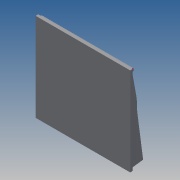
# Autodesk Inventor part: Bottom
Saved by Autodesk Inventor 2019 (Build 230136000, 136)
## iProperties
Created: 2022-10-28
Part Number: Bottom
Material: Generisch
Document SubType Name: Modeling
Designer: Dominik Schmidt
Density: 1 g/cm^3
Appearance: Vorgabe
Author: Dominik Schmidt
Autodesk Inventor part; units mm, degrees
ref_plane "YZ Plane" through (0, 0, 0) normal (1, 0, 0) x (0, 1, 0)
ref_plane "XZ Plane" through (0, 0, 0) normal (0, 1, 0) x (-1, 0, 0)
ref_plane "XY Plane" through (0, 0, 0) normal (0, 0, 1) x (1, 0, 0)
sketch "Skizze1" plane through (0, 0, 0) normal (0, 0, 1) x (1, 0, 0)
  line L0 (0, 0) -> (0, -76.060239)
  line L1 (0, -76.060239) -> (-35.95, -76.060239)
  line L2 (-45.45, -76.060239) -> (-81.4, -76.060239)
  line L3 (-81.4, -76.060239) -> (-81.4, 0)
  line L4 (-81.4, 0) -> (0, 0)
  line L5 (0, -76.060239) -> (-81.4, -76.060239)
  line L6 (-81.4, -76.060239) -> (-81.4, 0)
  line L7 (-81.4, 0) -> (0, 0)
  line L8 (0, 0) -> (0, -76.060239)
  constraints: 8 end point, 2 parallel, 1 horizontal, 1 perpendicular
extrude "Extrusion1" add sketch "Skizze1" along normal blind 2
sketch "Skizze2" plane through (0, 0, 0) normal (0, 0, -1) x (-1, 0, 0)
  point P0 (0, 0)
sketch "Skizze3" plane through (0, 0, 0) normal (0, 0, -1) x (-1, 0, 0)
  line L0 (35.95, -74.849731) -> (1.2, -74.849731)
  line L1 (80.2, -74.849731) -> (45.45, -74.849731)
  line L2 (49.95, -74.849731) -> (31.45, -74.849731)
  line L3 (31.45, -74.849731) -> (31.45, -50.349731)
  line L4 (31.45, -50.349731) -> (49.95, -50.349731)
  line L5 (49.95, -50.349731) -> (49.95, -74.849731)
  line L6 (81.4, 0) -> (81.4, -76.060239)
  line L7 (31.45, -50.349731) -> (29.45, -50.349731)
  line L8 (29.45, -50.349731) -> (29.45, -53.349731)
  line L9 (29.45, -53.349731) -> (31.45, -53.349731)
  line L10 (31.45, -53.349731) -> (31.45, -50.349731)
  line L11 (49.95, -50.349731) -> (51.95, -50.349731)
  line L12 (51.95, -50.349731) -> (51.95, -53.349731)
  line L13 (51.95, -53.349731) -> (49.95, -53.349731)
  line L14 (49.95, -53.349731) -> (49.95, -50.349731)
  line L15 (31.45, -50.349731) -> (34.45, -50.349731)
  line L16 (34.45, -50.349731) -> (34.45, -48.349731)
  line L17 (34.45, -48.349731) -> (31.45, -48.349731)
  line L18 (31.45, -48.349731) -> (31.45, -50.349731)
  line L19 (49.95, -50.349731) -> (46.95, -50.349731)
  line L20 (46.95, -50.349731) -> (46.95, -48.349731)
  line L21 (46.95, -48.349731) -> (49.95, -48.349731)
  line L22 (49.95, -48.349731) -> (49.95, -50.349731)
  line L23 (51.95, -50.349731) -> (49.95, -50.349731)
  line L24 (49.95, -50.349731) -> (49.95, -48.349731)
  line L25 (49.95, -48.349731) -> (51.95, -48.349731)
  line L26 (51.95, -48.349731) -> (51.95, -50.349731)
  line L27 (31.45, -50.349731) -> (29.45, -50.349731)
  line L28 (29.45, -50.349731) -> (29.45, -48.349731)
  line L29 (29.45, -48.349731) -> (31.45, -48.349731)
  line L30 (31.45, -48.349731) -> (31.45, -50.349731)
  point P0 (0, 0)
  dimension "d2" = 18.5
  dimension "d3" = 24.5
  dimension "d4" = 31.45
  dimension "d5" = 2
  dimension "d6" = 3
  dimension "d7" = 2
  dimension "d8" = 3
  dimension "d9" = 3
  dimension "d10" = 2
  dimension "d11" = 3
  dimension "d12" = 2
  constraints: 56 end point, 14 parallel, 7 horizontal, 7 perpendicular, 2 point on line
  measures "d2" distance of L3.end L4.end
  measures "d3" distance of L2.end L3.end
  measures "d4" distance between parallel lines of L6 L5
  measures "d5" distance of L9.end L8.end
  measures "d6" distance of L8.end L7.end
  measures "d7" distance of L12.end L13.end
  measures "d8" distance of L11.end L12.end
  measures "d9" distance of L17.end L16.end
  measures "d10" distance of L16.end L15.end
  measures "d11" distance of L20.end L21.end
  measures "d12" distance of L19.end L20.end
extrude "Extrusion2" add sketch "Skizze3" along normal blind 5 contours L9 L8 L7 L3 | L18 L17 L16 L4 | L7 L28 L29 L18 | L5 L11 L12 L13 | L22 L25 L26 L11 | L4 L20 L21 L22
sketch "Skizze4" plane through (-29.45, -53.349731, 0) normal (1, 0, 0) x (0, 0, -1)
  line L0 (9.128291, -19.280595) -> (0.713908, 44.163855)
  line L1 (0, -22.710508) -> (0, 53.349731)
  line L2 (5.628953, 7.104417) -> (6.752463, -1.366854)
  line L3 (6.752463, -1.366854) -> (5.208439, -1.571632)
  line L4 (5.208439, -1.571632) -> (4.084928, 6.899639)
  line L5 (4.084928, 6.899639) -> (5.628953, 7.104417)
  line L6 (5.628953, 7.104417) -> (6.752463, -1.366854)
  line L7 (6.752463, -1.366854) -> (5.208439, -1.571632)
  line L8 (5.208439, -1.571632) -> (4.084928, 6.899639)
  line L9 (4.084928, 6.899639) -> (5.628953, 7.104417)
  line L10 (5.628953, 7.104417) -> (6.752463, -1.366854)
  line L11 (6.752463, -1.366854) -> (4.791633, -1.626911)
  line L12 (4.791633, -1.626911) -> (3.668123, 6.84436)
  line L13 (3.668123, 6.84436) -> (5.628953, 7.104417)
  dimension "d17" = 1.978
  constraints: 24 end point, 6 parallel, 3 perpendicular, 2 collinear, 2 point on line
  measures "d17" distance of L2.end L11.end
extrude "Extrusion4" cut sketch "Skizze4" against normal blind 38.25
sketch "Skizze5" plane through (-51.95, -53.349731, 0) normal (-1, 0, 0) x (0, 0, 1)
  line L0 (-3.912733, 5) -> (-4.575863, 0)
  line L1 (0, 0) -> (-4.575863, 0)
  line L2 (0, 5) -> (0, 0)
  line L3 (0, 5) -> (-3.912733, 5)
  point P0 (0, 53.349731)
extrude "Extrusion5" add sketch "Skizze5" along normal blind 20
sketch "Skizze6" plane through (-71.95, -53.349731, 0) normal (-1, 0, 0) x (0, 0, 1)
  line L0 (-6.49237, -14.450462) -> (-0.576826, 30.152737)
  line L1 (-4.575863, 0) -> (-4.177985, 3)
  line L2 (-0.576826, 30.152737) -> (0, 30.076234)
  line L3 (0, -22.710508) -> (0, 53.349731)
  line L4 (-6.49237, -14.450462) -> (0, -14.450462)
  line L5 (-5.553925, -7.374589) -> (0, -7.374589)
  line L6 (0, -14.450462) -> (0, -7.374589)
  line L7 (-2.560597, 15.195102) -> (0, 15.195102)
  line L8 (0, 15.195102) -> (0, 30.076234)
  constraints: 14 end point, 6 point on line, 4 perpendicular, 1 collinear, 1 horizontal, 1 parallel
extrude "Extrusion6" add sketch "Skizze6" against normal up to surface (42.5 mm away) contours L0 L5 L3 L4 | L7 L0 L2 L3
sketch "Skizze8" plane through (0, 0, 0) normal (0, 0, -1) x (-1, 0, 0)
  line L0 (34.45, -50.349731) -> (31.45, -50.349731)
  line L1 (71.95, -67.800193) -> (29.45, -67.800193)
  line L2 (31.45, -50.349731) -> (49.95, -50.349731)
  line L3 (49.95, -50.349731) -> (49.95, -67.800193)
  line L4 (49.95, -67.800193) -> (31.45, -67.800193)
  line L5 (31.45, -67.800193) -> (31.45, -50.349731)
  point P0 (0, 0)
  dimension "d24" = 18.5
  constraints: 8 end point, 2 parallel, 1 horizontal, 1 perpendicular, 1 point on line
  measures "d24" distance of L3.end L4.end
sketch "Skizze9" plane through (0, 0, 0) normal (0, 0, -1) x (-1, 0, 0)
  line L0 (56.390705, -39.436288) -> (48.418409, -39.436288)
  line L1 (48.418409, -39.436288) -> (48.418409, -20.196482)
  line L2 (48.418409, -20.196482) -> (56.390705, -20.196482)
  line L3 (56.390705, -20.196482) -> (56.390705, -39.436288)
  point P0 (0, 0)
  constraints: 8 end point, 2 parallel, 1 horizontal, 1 perpendicular
extrude "Extrusion7" cut sketch "Skizze9" along normal blind 3
extrude "Extrusion8" cut sketch "Skizze8" along normal blind 7.25
sketch "Skizze10" plane through (0, 0, 0) normal (0, 0, -1) x (-1, 0, 0)
  line L0 (80.2, -1.210508) -> (80.2, -74.849731)
  line L1 (1.2, -74.849731) -> (1.2, -1.210508)
  line L2 (80.2, -70.638844) -> (78.2, -70.638844)
  line L3 (78.2, -70.638844) -> (78.2, -6.313614)
  line L4 (78.2, -6.313614) -> (80.2, -6.313614)
  line L5 (80.2, -6.313614) -> (80.2, -70.638844)
  line L6 (1.2, -70.638844) -> (3.2, -70.638844)
  line L7 (3.2, -70.638844) -> (3.2, -6.313614)
  line L8 (3.2, -6.313614) -> (1.2, -6.313614)
  line L9 (1.2, -6.313614) -> (1.2, -70.638844)
  point P0 (0, 0)
  dimension "d29" = 2
  dimension "d30" = 2
  constraints: 16 end point, 4 parallel, 4 point on line, 2 horizontal, 2 perpendicular
  measures "d29" distance of L3.end L4.end
  measures "d30" distance of L8.end L7.end
extrude "Extrusion9" add sketch "Skizze10" along normal blind 5
sketch "Skizze11" plane through (-1.2, -70.638844, 0) normal (1, 0, 0) x (0, 0, -1)
  line L0 (0, 64.32523) -> (5, 64.32523)
  line L1 (1.333936, 64.32523) -> (5, 44.186953)
  line L2 (5, 0) -> (5, 64.32523)
  line L3 (5, 64.32523) -> (1.333936, 64.32523)
  line L4 (5, 0) -> (5, 64.32523)
  line L5 (5, 44.186953) -> (5, 64.32523)
  point P0 (0, 70.638844)
  constraints: 6 end point, 2 point on line, 1 horizontal, 1 vertical
extrude "Extrusion10" cut sketch "Skizze11" against normal blind 79
sketch "Skizze12" plane through (0, 0, 0) normal (0, 0, -1) x (-1, 0, 0)
  line L0 (1.2, -1.210508) -> (80.2, -1.210508)
  line L1 (67.433498, -1.210508) -> (17.433498, -1.210508)
  line L2 (17.433498, -1.210508) -> (17.433498, -3.210508)
  line L3 (17.433498, -3.210508) -> (67.433498, -3.210508)
  line L4 (67.433498, -3.210508) -> (67.433498, -1.210508)
  point P0 (0, 0)
  dimension "d35" = 50
  dimension "d36" = 2
  constraints: 8 end point, 2 parallel, 1 horizontal, 1 perpendicular, 1 point on line
  measures "d35" distance of L3.end L2.end
  measures "d36" distance of L2.end L1.end
extrude "Extrusion11" add sketch "Skizze12" along normal blind 2
sketch "Skizze13" plane through (0, -76.060239, 0) normal (1, 0, 0) x (0, 0, -1)
  line L0 (0, 76.060239) -> (5.947917, 76.849088)
  line L1 (0, 76.060239) -> (-2, 76.060239)
  line L2 (0, 76.060239) -> (-5.27108, 75.379971)
  line L3 (-5.27108, 75.379971) -> (-3.751939, 78.131622)
  line L4 (-3.751939, 78.131622) -> (0, 76.060239)
  constraints: 6 end point, 1 perpendicular
extrude "Extrusion12" cut sketch "Skizze13" against normal up to surface (81.4 mm away)
sketch "Skizze14" plane through (0, -76.060239, 2) normal (1, 0, 0) x (0, 0, -1)
  line L0 (17.861112, 2.103596) -> (2, 0)
  line L1 (2, 0) -> (0, 0)
  line L2 (2, 0) -> (0, -0.265252)
  line L3 (0, -0.265252) -> (0, 0)
  line L4 (0, 0) -> (2, 0)
  point P0 (2, 76.060239)
  constraints: 6 end point, 2 perpendicular
extrude "Extrusion13" add sketch "Skizze14" against normal up to surface (81.4 mm away)
sketch "Skizze15" plane through (-1.2, -70.638844, 0) normal (1, 0, 0) x (0, 0, -1)
  line L0 (13.225044, -2.456903) -> (3.627388, 69.909422)
  line L1 (1.333936, 64.32523) -> (5, 44.186953)
  line L2 (1.333936, 64.32523) -> (10.003979, -1.046893)
  line L3 (10.003979, -1.046893) -> (0, -1.046893)
  line L4 (0, -1.046893) -> (0, 64.32523)
  line L5 (0, 64.32523) -> (1.333936, 64.32523)
  point P0 (0, 70.638844)
  constraints: 8 end point, 2 perpendicular, 1 horizontal, 1 parallel
extrude "Extrusion14" add sketch "Skizze15" against normal up to surface (2 mm away)
sketch "Skizze16" plane through (-80.2, -70.638844, 0) normal (-1, 0, 0) x (0, 0, 1)
  line L0 (0, -1.046893) -> (-10.003979, -1.046893)
  line L1 (-10.003979, -1.046893) -> (-5, 36.68311)
  line L2 (0, 64.32523) -> (0, -1.046893)
  line L3 (0, 64.32523) -> (-1.333936, 64.32523)
  line L4 (-5, 44.186953) -> (-5, 0)
  line L5 (-5, 36.054624) -> (-1.333936, 64.32523)
  point P0 (0, 70.638844)
  constraints: 2 end point, 2 point on line
extrude "Extrusion15" add sketch "Skizze16" against normal up to surface (2 mm away)
sketch "Skizze17" plane through (-1.2, -71.685737, 0) normal (1, 0, 0) x (0, 0, -1)
  line L0 (13.225044, -1.41001) -> (0, -3.163995)
  line L1 (10.003979, 0) -> (0, 0)
  line L2 (10.003979, 0) -> (10.003979, -1.837207)
  line L3 (0, 0) -> (0, -3.163995)
  line L4 (0, -4.374503) -> (0, 71.685737)
  constraints: 4 end point, 1 collinear, 1 point on line, 1 vertical
extrude "Extrusion16" add sketch "Skizze17" against normal blind 4.75
sketch "Skizze18" plane through (-80.2, -71.685737, -10.003979) normal (-1, 0, 0) x (0, 0, 1)
  line L0 (0, -1.837207) -> (10.003979, -3.163995)
  line L1 (10.003979, 0) -> (10.003979, -3.163995)
  line L2 (10.003979, 0) -> (0, 0)
  line L3 (0, 0) -> (0, -1.837207)
  line L4 (10.003979, 0) -> (0, 0)
  line L5 (2.164528, 0) -> (2.164528, -2.12428)
  point P0 (10.003979, 71.685737)
  constraints: 2 end point, 2 point on line, 1 perpendicular
extrude "Extrusion17" add sketch "Skizze18" against normal blind 27.25 contours L5 L2 L1 L0
fillet "Rundung2" radius 2 1 edges at (-79.2, -71.6857, -10.004)
fillet "Rundung3" radius 40 4 edges at (-2.2, -26.4519, -5) (-2.2, -33.9557, -5) (-79.2, -33.9557, -5) (-79.2, -26.4519, -5)
sketch "Skizze19" plane through (-17.433498, -3.210508, 0) normal (1, 0, 0) x (0, 0, -1)
  line L0 (0, 0) -> (0, 2) projected
  line L1 (0, 0) -> (2, 0) projected
  line L2 (2, 2) -> (2, 0) projected
  line L3 (0, 2) -> (2, 2) projected
  point P0 (0, 3.210508)
extrude "Extrusion18" add sketch "Skizze19" along normal up to surface (16.233498 mm away)
sketch "Skizze20" plane through (-67.433498, -3.210508, 0) normal (-1, 0, 0) x (0, 0, 1)
  line L0 (0, 2) -> (0, 0) projected
  line L1 (0, 2) -> (-2, 2) projected
  line L2 (-2, 0) -> (-2, 2) projected
  line L3 (0, 0) -> (-2, 0) projected
  point P0 (0, 3.210508)
extrude "Extrusion19" add sketch "Skizze20" along normal up to surface (12.766502 mm away)
sketch "Skizze21" plane through (-78.2, -71.685737, 0) normal (1, 0, 0) x (0, 0, -1)
  arc A0 (5, 41.62263) -> (4.353228, 48.786671) centre (-35, 41.62263) ccw
  line L0 (4.353228, 48.786671) -> (1.333936, 65.372123)
  line L1 (0, 65.372123) -> (1.333936, 65.372123)
  line L2 (0, 0) -> (0, 65.372123)
  line L3 (7.839451, 0) -> (0, 0)
  arc A1 (7.839451, 0) -> (9.704314, 2.259479) centre (7.721674, 1.996529) ccw
  line L4 (5.347219, 35.11197) -> (9.704314, 2.259479)
  arc A2 (5, 40.37096) -> (5.347219, 35.11197) centre (45, 40.37096) ccw
  line L5 (5, 41.62263) -> (5, 40.37096)
  point P0 (0, 71.685737)
extrude "Extrusion20" cut sketch "Skizze21" against normal blind 0.5
